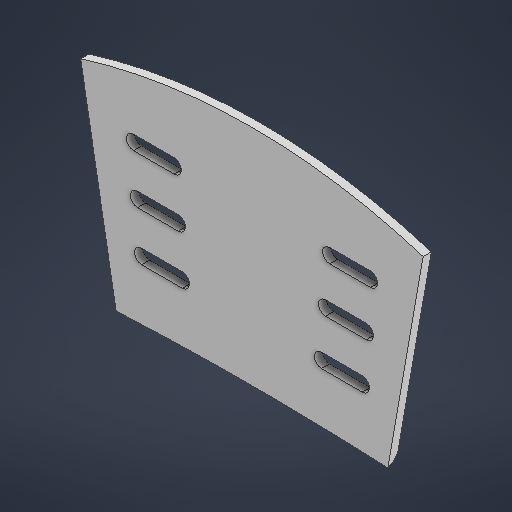
# Autodesk Inventor part: Double Shear Plate
Saved by Autodesk Inventor 2026 (Build 300175000, 175)
## iProperties
Created: 2025-11-03
Part Number: Double Shear Plate
Material: Generic
Document SubType Name: Sheet Metal
Designer: Brandon Portillo
Density: 1 g/cm^3
Sheet Metal Rule: Default
Appearance: Default
Author: Brandon Portillo
Autodesk Inventor part; units mm, degrees
ref_plane "YZ Plane" through (0, 0, 0) normal (1, 0, 0) x (0, 1, 0)
ref_plane "XZ Plane" through (0, 0, 0) normal (0, 1, 0) x (-1, 0, 0)
ref_plane "XY Plane" through (0, 0, 0) normal (0, 0, 1) x (1, 0, 0)
sketch "Sketch1" plane through (0, 0, 0) normal (0, 0, 1) x (1, 0, 0)
  line L0 (0, 0) -> (200, 0) construction
  arc A0 (200, 0) -> (0, 0) centre (100, -2022.5294) ccw
  line L1 (200, 0) -> (226.0472, 147.7212)
  line L2 (200, 0) -> (350, 0) construction
  line L3 (100, 2.4706) -> (100, 110.946)
  line L4 (0, 0) -> (-26.0472, 147.7212)
  arc A1 (226.0472, 147.7212) -> (-26.0472, 147.7212) centre (100, -252.9184) ccw
  dimension "d4" = 2025
  dimension "d5" = 150
  dimension "d6" = 80
  dimension "d7" = 420
  dimension "d20" = 200
  measures "d4" radius of A0
  measures "d5" distance of L0.end L1.end
  measures "d6" angle of L2 L1
  measures "d7" radius of A1
  measures "d20" distance of L0.end L0.start
extrude "Plate1" add sketch "Sketch1" along normal blind 6
sketch "Sketch2" plane through (0, 0, 6) normal (0, 0, 1) x (1, 0, 0)
  arc A0 (200, 0) -> (0, 0) centre (100, -2022.5294) ccw projected
  line L0 (100, 2.4706) -> (100, 167.0816)
  arc A1 (226.0472, 147.7212) -> (-26.0472, 147.7212) centre (100, -252.9184) ccw projected
  arc A2 (100, 2.4706) -> (0, 0) centre (100, -2022.5294) ccw
  arc A3 (100, 167.0816) -> (-26.0472, 147.7212) centre (100, -252.9184) ccw
  line L1 (45.7974, 79.0021) -> (15.7974, 79.0021) construction
  line L2 (45.7974, 84.2521) -> (15.7974, 84.2521)
  line L3 (15.7974, 73.7521) -> (45.7974, 73.7521)
  arc A4 (45.7974, 73.7521) -> (45.7974, 84.2521) centre (45.7974, 79.0021) ccw
  arc A5 (15.7974, 84.2521) -> (15.7974, 73.7521) centre (15.7974, 79.0021) ccw
  line L4 (30.7974, 79.0021) -> (27.8022, 113.8737)
  line L5 (30.7974, 79.0021) -> (33.7926, 44.1305)
  line L6 (18.7926, 44.1305) -> (48.7926, 44.1305) construction
  line L7 (18.7926, 38.8805) -> (48.7926, 38.8805)
  line L8 (48.7926, 49.3805) -> (18.7926, 49.3805)
  arc A6 (18.7926, 49.3805) -> (18.7926, 38.8805) centre (18.7926, 44.1305) ccw
  arc A7 (48.7926, 38.8805) -> (48.7926, 49.3805) centre (48.7926, 44.1305) ccw
  line L9 (33.7926, 44.1305) -> (63.7926, 44.1305) construction
  line L10 (12.8022, 113.8737) -> (42.8022, 113.8737) construction
  line L11 (12.8022, 108.6237) -> (42.8022, 108.6237)
  line L12 (42.8022, 119.1237) -> (12.8022, 119.1237)
  arc A8 (12.8022, 119.1237) -> (12.8022, 108.6237) centre (12.8022, 113.8737) ccw
  arc A9 (42.8022, 108.6237) -> (42.8022, 119.1237) centre (42.8022, 113.8737) ccw
  line L13 (154.2026, 79.0021) -> (184.2026, 79.0021) construction
  line L14 (154.2026, 84.2521) -> (184.2026, 84.2521)
  line L15 (184.2026, 73.7521) -> (154.2026, 73.7521)
  arc A10 (154.2026, 84.2521) -> (154.2026, 73.7521) centre (154.2026, 79.0021) ccw
  arc A11 (184.2026, 73.7521) -> (184.2026, 84.2521) centre (184.2026, 79.0021) ccw
  line L16 (169.2026, 79.0021) -> (172.1978, 113.8737)
  line L17 (169.2026, 79.0021) -> (166.2074, 44.1305)
  line L18 (181.2074, 44.1305) -> (151.2074, 44.1305) construction
  line L19 (181.2074, 38.8805) -> (151.2074, 38.8805)
  line L20 (151.2074, 49.3805) -> (181.2074, 49.3805)
  arc A12 (181.2074, 38.8805) -> (181.2074, 49.3805) centre (181.2074, 44.1305) ccw
  arc A13 (151.2074, 49.3805) -> (151.2074, 38.8805) centre (151.2074, 44.1305) ccw
  line L21 (187.1978, 113.8737) -> (157.1978, 113.8737) construction
  line L22 (187.1978, 108.6237) -> (157.1978, 108.6237)
  line L23 (157.1978, 119.1237) -> (187.1978, 119.1237)
  arc A14 (187.1978, 108.6237) -> (187.1978, 119.1237) centre (187.1978, 113.8737) ccw
  arc A15 (157.1978, 119.1237) -> (157.1978, 108.6237) centre (157.1978, 113.8737) ccw
  dimension "d9" = 15
  dimension "d10" = 10.5
  dimension "d11" = 35
  dimension "d12" = 35
  dimension "d13" = 15
  dimension "d14" = 0
  dimension "d15" = 10.5
  dimension "d16" = 15
  dimension "d17" = 10.5
  constraints: 60 end point, 30 point on circle, 21 symmetric about line, 14 centre point, 12 tangent, 4 horizontal, 3 midpoint, 3 parallel, 2 concentric, 1 collinear, 1 vertical, 6 other
  measures "d9" distance of L4.start L1.end
  measures "d10" diameter of A5
  measures "d11" distance of L4.start L4.end
  measures "d12" distance of L4.start L5.end
  measures "d13" distance of L5.end L6.end
  measures "d14" distance between parallel lines of L6 L9
  measures "d15" diameter of A7
  measures "d16" distance of L4.end L10.end
  measures "d17" diameter of A9
extrude "Cut1" cut sketch "Sketch2" against normal blind 6
fillet "Fillet1" radius 10 1 edges at (100, 2.4706, 0)
equation "\"d18\" = Thickness"
equation "\"d8\" = Thickness"
equation "\"BendRadius\" = Thickness"
equation "\"BendReliefWidth\" = Thickness"
equation "\"BendReliefDepth\" = 0.5 * Thickness"
equation "\"CornerReliefSize\" = 4 * Thickness"
equation "\"MinimumRemnant\" = 2 * Thickness"
equation "\"TransitionRadius\" = BendRadius"
equation "\"JacobiRadiusSize\" = BendRadius"
equation "\"GapSize\" = Thickness"
equation "\"Thickness\" = 6"
body "Solid1"
